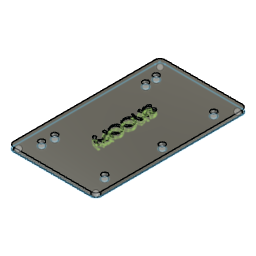
lidar mount int round (Autodesk Fusion 360 design; units mm, degrees)
Autodesk Fusion 360 part; units mm, degrees
note: some values were not read from the file. Set by a fixed rule: which sketch regions a step uses.
sketch "Sketch1" plane through (0, 0, 0) normal (0, 0, 1) x (1, 0, 0)
  circle A0 centre (87.3491, 70.8587) radius 1.5
  circle A1 centre (87.3491, 11.8587) radius 1.5
  circle A2 centre (118.3596, 69.4087) radius 1.5
  circle A3 centre (118.3596, 13.3087) radius 1.5
  line L0 (80.1858, 77.5) -> (80.1858, 4.6534)
  line L1 (82.6858, 2.1534) -> (122.5, 2.1534)
  line L2 (125, 4.6534) -> (125, 77.5)
  line L3 (122.5, 80) -> (82.6858, 80)
  line L4 (80.1858, 80) -> (80.1858, 79.4159)
  circle A4 centre (87.7805, 65) radius 1.5
  circle A5 centre (87.7805, 18.2) radius 1.5
  circle A6 centre (119.7005, 41.6) radius 1.5
  line L5 (103.1596, 52.1892) -> (102.3232, 52.8089)
  spline S0 degree 2 poles (102.3232, 52.8089) (102.9092, 53.3034) (102.9092, 54.1336) knots 0 0 0 1 1 1
  spline S1 degree 2 poles (102.9092, 54.1336) (102.9092, 54.326) (102.8787, 54.4572) knots 0 0 0 1 1 1
  spline S2 degree 2 poles (102.8787, 54.4572) (103.1168, 54.21) (103.3549, 53.9597) knots 0 0 0 1 1 1
  spline S3 degree 2 poles (103.3549, 53.9597) (103.5167, 53.7338) (103.5167, 53.3522) knots 0 0 0 1 1 1
  spline S4 degree 2 poles (103.5167, 53.3522) (103.5167, 52.7325) (103.1596, 52.1892) knots 0 0 0 1 1 1
  spline S5 degree 2 poles (99.927, 51.7527) (99.2401, 51.7527) (98.7853, 52.4639) knots 0 0 0 1 1 1
  spline S6 degree 2 poles (98.7853, 52.4639) (98.3793, 53.0836) (98.3793, 53.8009) knots 0 0 0 1 1 1
  spline S7 degree 2 poles (98.3793, 53.8009) (98.5594, 53.459) (98.8219, 53.2026) knots 0 0 0 1 1 1
  spline S8 degree 2 poles (98.8219, 53.2026) (99.1608, 52.8699) (99.466, 52.8699) knots 0 0 0 1 1 1
  spline S9 degree 2 poles (99.466, 52.8699) (99.8537, 52.8699) (100.223, 53.6971) knots 0 0 0 1 1 1
  spline S10 degree 2 poles (100.223, 53.6971) (100.5588, 54.4572) (100.8976, 55.2264) knots 0 0 0 1 1 1
  spline S11 degree 2 poles (100.8976, 55.2264) (101.3586, 56.0476) (101.9782, 56.0476) knots 0 0 0 1 1 1
  spline S12 degree 2 poles (101.9782, 56.0476) (102.43, 56.0476) (102.8726, 55.4157) knots 0 0 0 1 1 1
  spline S13 degree 2 poles (102.8726, 55.4157) (103.2359, 54.9029) (103.3793, 54.3656) knots 0 0 0 1 1 1
  spline S14 degree 2 poles (103.3793, 54.3656) (102.9154, 55.0525) (102.4788, 55.0525) knots 0 0 0 1 1 1
  spline S15 degree 2 poles (102.4788, 55.0525) (102.1217, 55.0525) (101.6608, 54.1947) knots 0 0 0 1 1 1
  spline S16 degree 2 poles (101.6608, 54.1947) (101.2609, 53.401) (100.861, 52.6074) knots 0 0 0 1 1 1
  spline S17 degree 2 poles (100.861, 52.6074) (100.3665, 51.7527) (99.927, 51.7527) knots 0 0 0 1 1 1
  spline S18 degree 2 poles (98.8403, 53.5201) (98.6724, 53.7887) (98.4953, 54.0512) knots 0 0 0 1 1 1
  spline S19 degree 2 poles (98.4953, 54.0512) (98.3091, 54.3717) (98.3091, 54.6465) knots 0 0 0 1 1 1
  spline S20 degree 2 poles (98.3091, 54.6465) (98.3091, 55.0586) (98.5655, 55.608) knots 0 0 0 1 1 1
  spline S21 degree 2 poles (98.5655, 55.608) (98.7853, 56.072) (99.0906, 56.478) knots 0 0 0 1 1 1
  line L6 (99.0906, 56.478) -> (100.0521, 55.666)
  spline S22 degree 2 poles (100.0521, 55.666) (99.5332, 55.3394) (99.1974, 54.8205) knots 0 0 0 1 1 1
  spline S23 degree 2 poles (99.1974, 54.8205) (98.8342, 54.2588) (98.8342, 53.6849) knots 0 0 0 1 1 1
  spline S24 degree 2 poles (98.8342, 53.6849) (98.8342, 53.6025) (98.8403, 53.5201) knots 0 0 0 1 1 1
  spline S25 degree 2 poles (101.847, 46.4078) (100.1895, 46.4078) (98.3152, 47.2075) knots 0 0 0 1 1 1
  line L7 (98.3152, 47.2075) -> (98.4709, 47.6471)
  spline S26 degree 2 poles (98.4709, 47.6471) (99.2401, 47.3144) (100.2047, 47.3144) knots 0 0 0 1 1 1
  spline S27 degree 2 poles (100.2047, 47.3144) (101.4105, 47.3144) (102.4178, 47.7081) knots 0 0 0 1 1 1
  spline S28 degree 2 poles (102.4178, 47.7081) (102.5216, 47.9462) (102.5216, 48.2454) knots 0 0 0 1 1 1
  spline S29 degree 2 poles (102.5216, 48.2454) (102.5216, 49.1703) (101.792, 50.2844) knots 0 0 0 1 1 1
  line L8 (101.792, 50.2844) -> (102.2926, 50.2539)
  spline S30 degree 2 poles (102.2926, 50.2539) (102.8848, 49.5915) (103.2725, 48.7338) knots 0 0 0 1 1 1
  spline S31 degree 2 poles (103.2725, 48.7338) (103.6907, 47.815) (103.7243, 46.9908) knots 0 0 0 1 1 1
  spline S32 degree 2 poles (103.7243, 46.9908) (103.0863, 46.4078) (101.847, 46.4078) knots 0 0 0 1 1 1
  line L9 (98.5961, 50.0341) -> (98.0954, 51.2155)
  spline S33 degree 2 poles (98.0954, 51.2155) (98.883, 51.4352) (100.0399, 51.4352) knots 0 0 0 1 1 1
  spline S34 degree 2 poles (100.0399, 51.4352) (102.0088, 51.4352) (103.6907, 50.6294) knots 0 0 0 1 1 1
  line L10 (103.6907, 50.6294) -> (103.4404, 50.315)
  spline S35 degree 2 poles (103.4404, 50.315) (102.4972, 50.6019) (101.267, 50.6019) knots 0 0 0 1 1 1
  spline S36 degree 2 poles (101.267, 50.6019) (99.7469, 50.6019) (98.5961, 50.0341) knots 0 0 0 1 1 1
  spline S37 degree 2 poles (101.3464, 39.8449) (100.4733, 39.8449) (99.6644, 40.4493) knots 0 0 0 1 1 1
  spline S38 degree 2 poles (99.6644, 40.4493) (98.8983, 41.0201) (98.535, 41.8504) knots 0 0 0 1 1 1
  spline S39 degree 2 poles (98.535, 41.8504) (99.6278, 40.9194) (100.8793, 40.9194) knots 0 0 0 1 1 1
  spline S40 degree 2 poles (100.8793, 40.9194) (101.7523, 40.9194) (102.4758, 41.5573) knots 0 0 0 1 1 1
  spline S41 degree 2 poles (102.4758, 41.5573) (103.1992, 42.1953) (103.1992, 43.05) knots 0 0 0 1 1 1
  spline S42 degree 2 poles (103.1992, 43.05) (103.1992, 43.34) (103.0985, 43.6208) knots 0 0 0 1 1 1
  line L11 (103.0985, 43.6208) -> (103.6602, 43.0317)
  spline S43 degree 2 poles (103.6602, 43.0317) (103.6907, 42.7753) (103.6907, 42.5311) knots 0 0 0 1 1 1
  spline S44 degree 2 poles (103.6907, 42.5311) (103.6907, 41.4627) (103.0619, 40.6813) knots 0 0 0 1 1 1
  spline S45 degree 2 poles (103.0619, 40.6813) (102.3903, 39.8449) (101.3464, 39.8449) knots 0 0 0 1 1 1
  line L12 (99.0906, 41.945) -> (98.4404, 42.351)
  spline S46 degree 2 poles (98.4404, 42.351) (98.3274, 42.8821) (98.3274, 43.3644) knots 0 0 0 1 1 1
  spline S47 degree 2 poles (98.3274, 43.3644) (98.3274, 44.503) (98.9349, 45.2387) knots 0 0 0 1 1 1
  spline S48 degree 2 poles (98.9349, 45.2387) (99.5851, 46.0323) (100.7023, 46.0323) knots 0 0 0 1 1 1
  spline S49 degree 2 poles (100.7023, 46.0323) (101.6211, 46.0323) (102.5002, 45.2951) knots 0 0 0 1 1 1
  spline S50 degree 2 poles (102.5002, 45.2951) (103.3793, 44.5579) (103.5045, 43.6514) knots 0 0 0 1 1 1
  spline S51 degree 2 poles (103.5045, 43.6514) (103.0344, 44.2527) (102.3964, 44.5824) knots 0 0 0 1 1 1
  spline S52 degree 2 poles (102.3964, 44.5824) (101.7401, 44.9273) (101.0045, 44.9273) knots 0 0 0 1 1 1
  spline S53 degree 2 poles (101.0045, 44.9273) (100.0582, 44.9273) (99.4904, 44.3305) knots 0 0 0 1 1 1
  spline S54 degree 2 poles (99.4904, 44.3305) (98.9227, 43.7338) (98.9227, 42.7814) knots 0 0 0 1 1 1
  spline S55 degree 2 poles (98.9227, 42.7814) (98.9227, 42.238) (99.0906, 41.945) knots 0 0 0 1 1 1
  spline S56 degree 2 poles (101.3464, 33.3064) (100.4733, 33.3064) (99.6644, 33.9108) knots 0 0 0 1 1 1
  spline S57 degree 2 poles (99.6644, 33.9108) (98.8983, 34.4816) (98.535, 35.3119) knots 0 0 0 1 1 1
  spline S58 degree 2 poles (98.535, 35.3119) (99.6278, 34.3809) (100.8793, 34.3809) knots 0 0 0 1 1 1
  spline S59 degree 2 poles (100.8793, 34.3809) (101.7523, 34.3809) (102.4758, 35.0189) knots 0 0 0 1 1 1
  spline S60 degree 2 poles (102.4758, 35.0189) (103.1992, 35.6568) (103.1992, 36.5115) knots 0 0 0 1 1 1
  spline S61 degree 2 poles (103.1992, 36.5115) (103.1992, 36.8015) (103.0985, 37.0824) knots 0 0 0 1 1 1
  line L13 (103.0985, 37.0824) -> (103.6602, 36.4932)
  spline S62 degree 2 poles (103.6602, 36.4932) (103.6907, 36.2368) (103.6907, 35.9926) knots 0 0 0 1 1 1
  spline S63 degree 2 poles (103.6907, 35.9926) (103.6907, 34.9242) (103.0619, 34.1428) knots 0 0 0 1 1 1
  spline S64 degree 2 poles (103.0619, 34.1428) (102.3903, 33.3064) (101.3464, 33.3064) knots 0 0 0 1 1 1
  line L14 (99.0906, 35.4065) -> (98.4404, 35.8125)
  spline S65 degree 2 poles (98.4404, 35.8125) (98.3274, 36.3437) (98.3274, 36.826) knots 0 0 0 1 1 1
  spline S66 degree 2 poles (98.3274, 36.826) (98.3274, 37.9645) (98.9349, 38.7002) knots 0 0 0 1 1 1
  spline S67 degree 2 poles (98.9349, 38.7002) (99.5851, 39.4938) (100.7023, 39.4938) knots 0 0 0 1 1 1
  spline S68 degree 2 poles (100.7023, 39.4938) (101.6211, 39.4938) (102.5002, 38.7567) knots 0 0 0 1 1 1
  spline S69 degree 2 poles (102.5002, 38.7567) (103.3793, 38.0195) (103.5045, 37.1129) knots 0 0 0 1 1 1
  spline S70 degree 2 poles (103.5045, 37.1129) (103.0344, 37.7142) (102.3964, 38.0439) knots 0 0 0 1 1 1
  spline S71 degree 2 poles (102.3964, 38.0439) (101.7401, 38.3888) (101.0045, 38.3888) knots 0 0 0 1 1 1
  spline S72 degree 2 poles (101.0045, 38.3888) (100.0582, 38.3888) (99.4904, 37.7921) knots 0 0 0 1 1 1
  spline S73 degree 2 poles (99.4904, 37.7921) (98.9227, 37.1953) (98.9227, 36.2429) knots 0 0 0 1 1 1
  spline S74 degree 2 poles (98.9227, 36.2429) (98.9227, 35.6996) (99.0906, 35.4065) knots 0 0 0 1 1 1
  spline S75 degree 2 poles (102.6345, 28.4499) (101.6425, 28.4499) (101.09, 29.6862) knots 0 0 0 1 1 1
  spline S76 degree 2 poles (101.09, 29.6862) (100.6779, 30.6172) (100.6473, 31.7741) knots 0 0 0 1 1 1
  line L15 (100.6473, 31.7741) -> (101.1113, 31.8046)
  line L16 (101.1113, 31.8046) -> (101.1113, 31.7008)
  spline S77 degree 2 poles (101.1113, 31.7008) (101.0961, 30.901) (101.4349, 30.3241) knots 0 0 0 1 1 1
  spline S78 degree 2 poles (101.4349, 30.3241) (101.8348, 29.6312) (102.5918, 29.6312) knots 0 0 0 1 1 1
  spline S79 degree 2 poles (102.5918, 29.6312) (102.7963, 29.6312) (102.955, 30.0311) knots 0 0 0 1 1 1
  spline S80 degree 2 poles (102.955, 30.0311) (103.0924, 30.3608) (103.0924, 30.6111) knots 0 0 0 1 1 1
  spline S81 degree 2 poles (103.0924, 30.6111) (103.0924, 31.1636) (102.7291, 31.7741) knots 0 0 0 1 1 1
  line L17 (102.7291, 31.7741) -> (103.0985, 31.8046)
  spline S82 degree 2 poles (103.0985, 31.8046) (103.3549, 31.5238) (103.5167, 30.9682) knots 0 0 0 1 1 1
  spline S83 degree 2 poles (103.5167, 30.9682) (103.6602, 30.4737) (103.6602, 30.0372) knots 0 0 0 1 1 1
  spline S84 degree 2 poles (103.6602, 30.0372) (103.6602, 29.4358) (103.4404, 29.0054) knots 0 0 0 1 1 1
  spline S85 degree 2 poles (103.4404, 29.0054) (103.1718, 28.4499) (102.6345, 28.4499) knots 0 0 0 1 1 1
  line L18 (98.8403, 31.8046) -> (98.1901, 32.9249)
  spline S86 degree 2 poles (98.1901, 32.9249) (98.9532, 33.0683) (99.7896, 33.0683) knots 0 0 0 1 1 1
  spline S87 degree 2 poles (99.7896, 33.0683) (101.9294, 33.0683) (103.7243, 32.3632) knots 0 0 0 1 1 1
  line L19 (103.7243, 32.3632) -> (103.4099, 31.9938)
  spline S88 degree 2 poles (103.4099, 31.9938) (102.7719, 32.2564) (101.8042, 32.2564) knots 0 0 0 1 1 1
  spline S89 degree 2 poles (101.8042, 32.2564) (100.3482, 32.2564) (98.8403, 31.8046) knots 0 0 0 1 1 1
  line L20 (101.2731, 26.423) -> (100.8793, 26.6611)
  spline S90 degree 2 poles (100.8793, 26.6611) (101.148, 27.3296) (101.8653, 27.873) knots 0 0 0 1 1 1
  spline S91 degree 2 poles (101.8653, 27.873) (102.5094, 28.3675) (103.2786, 28.5934) knots 0 0 0 1 1 1
  line L21 (103.2786, 28.5934) -> (103.7914, 27.4059)
  spline S92 degree 2 poles (103.7914, 27.4059) (103.0863, 27.3296) (102.4422, 27.1098) knots 0 0 0 1 1 1
  spline S93 degree 2 poles (102.4422, 27.1098) (101.6302, 26.8351) (101.2731, 26.423) knots 0 0 0 1 1 1
  spline S94 degree 2 poles (103.5777, 24.7472) (101.9355, 24.8724) (100.4611, 25.5805) knots 0 0 0 1 1 1
  spline S95 degree 2 poles (100.4611, 25.5805) (98.7853, 26.3803) (98.0344, 27.6349) knots 0 0 0 1 1 1
  line L22 (98.0344, 27.6349) -> (99.1089, 28.4041)
  spline S96 degree 2 poles (99.1089, 28.4041) (99.811, 27.122) (101.0106, 26.2368) knots 0 0 0 1 1 1
  spline S97 degree 2 poles (101.0106, 26.2368) (102.311, 25.2722) (103.6724, 25.1929) knots 0 0 0 1 1 1
  line L23 (103.6724, 25.1929) -> (103.5777, 24.7472)
  arc A7 (82.6858, 80) -> (80.1858, 77.5) centre (82.6858, 77.5) ccw
  arc A8 (125, 77.5) -> (122.5, 80) centre (122.5, 77.5) ccw
  arc A9 (80.1858, 4.6534) -> (82.6858, 2.1534) centre (82.6858, 4.6534) ccw
  arc A10 (122.5, 2.1534) -> (125, 4.6534) centre (122.5, 4.6534) ccw
  dimension "d53" = 3
  dimension "d61" = 3
  dimension "d78" = 3
  dimension "d79" = 46.8
  dimension "d80" = 3
  dimension "d83" = 3
  dimension "d89" = 2.5
  constraint perpendicular L0 L1
  constraint perpendicular L2 L3
  constraint perpendicular L3 L4
  constraint coincident L4.start L3
  constraint coincident L4.end L0
  constraint tangent L3 A7
  constraint tangent L0 A7
  constraint tangent L3 A8
  constraint tangent L2 A8
  constraint equal A7 A8
  constraint tangent L0 A9
  constraint tangent L1 A9
  constraint equal A7 A9
  constraint tangent L2 A10
  constraint tangent L1 A10
  constraint equal A7 A10
  measures "d53" diameter of A0
  measures "d61" diameter of A2
  measures "d78" diameter of A4
  measures "d79" distance of A4.centre A5.centre
  measures "d80" diameter of A5
  measures "d83" diameter of A6
  measures "d89" radius of A7
extrude "Extrude3" add sketch "Sketch1" along normal blind 2
